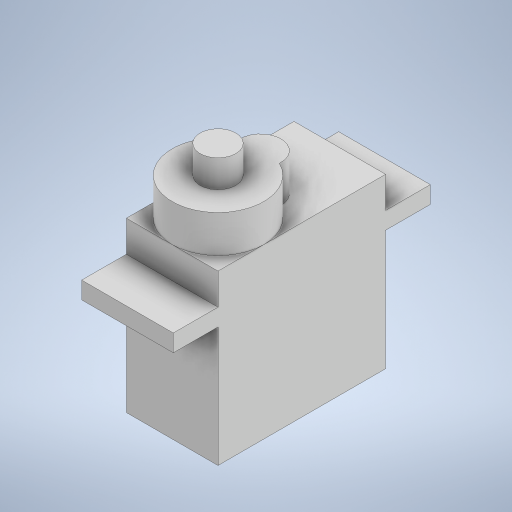
# Autodesk Inventor part: servomoteur
Saved by Autodesk Inventor 2024.1 (Build 281209000, 209)
## iProperties
Created: 2024-04-06
Part Number: servomoteur
Material: Générique
Document SubType Name: Modeling
Designer: chass
Density: 1 g/cm^3
Appearance: Par défaut
Author: chass
Autodesk Inventor part; units mm, degrees
ref_plane "YZ Plane" through (0, 0, 0) normal (1, 0, 0) x (0, 1, 0)
ref_plane "XZ Plane" through (0, 0, 0) normal (0, 1, 0) x (-1, 0, 0)
ref_plane "XY Plane" through (0, 0, 0) normal (0, 0, 1) x (1, 0, 0)
sketch "Esquisse1" plane through (0, 0, 0) normal (0, 1, 0) x (-1, 0, 0)
  line L0 (6.15, 11.25) -> (-6.15, 11.25)
  line L1 (-6.15, 11.25) -> (-6.15, -11.25)
  line L2 (-6.15, -11.25) -> (6.15, -11.25)
  line L3 (6.15, -11.25) -> (6.15, 11.25)
  line L4 (6.15, 11.25) -> (-6.15, -11.25)
  line L5 (-6.15, 11.25) -> (6.15, -11.25)
  point P0 (0, 0)
  point P1 (0, 0)
  point P2 (0, 0)
  dimension "d0" = 22.5
  dimension "d1" = 12.3
  constraints: 12 end point, 2 midpoint, 2 parallel, 1 coincident, 1 horizontal, 1 perpendicular
  measures "d0" distance of L2.end L0.start
  measures "d1" distance of L1.end L2.end
extrude "Extrusion1" add sketch "Esquisse1" along normal blind 22.6
sketch "Esquisse2" plane through (-6.15, 0, 11.25) normal (0, 0, 1) x (1, 0, 0)
  line L0 (0, 0) -> (0, 22.6) projected
  line L1 (12.3, 0) -> (12.3, 22.6) projected
  line L2 (0, 18.4) -> (12.3, 18.4)
  line L3 (12.3, 18.4) -> (12.3, 16.1)
  line L4 (12.3, 16.1) -> (0, 16.1)
  line L5 (0, 16.1) -> (0, 18.4)
  line L6 (0, 0) -> (12.3, 0) projected
  point P0 (6.15, 0)
  point P1 (0, 16.1)
  dimension "d4" = 2.3
  dimension "d5" = 16.1
  constraints: 8 end point, 2 parallel, 2 point on line, 1 horizontal, 1 perpendicular
  measures "d4" distance between parallel lines of L4 L2
  measures "d5" distance between parallel lines of L4 L6
extrude "Extrusion2" add sketch "Esquisse2" along normal blind 6 contours L0 L2 L1 L4
sketch "Esquisse3" plane through (6.15, 0, -11.25) normal (0, 0, -1) x (-1, 0, 0)
  line L0 (12.3, 18.4) -> (0, 18.4) projected
  line L1 (12.3, 0) -> (12.3, 16.1) projected
  line L2 (0, 18.4) -> (12.3, 18.4)
  line L3 (12.3, 18.4) -> (12.3, 16.1)
  line L4 (12.3, 16.1) -> (0, 16.1)
  line L5 (0, 16.1) -> (0, 18.4)
  point P0 (6.15, 0)
  constraints: 8 end point, 2 parallel, 1 horizontal, 1 perpendicular
extrude "Extrusion3" add sketch "Esquisse3" along normal blind 6
sketch "Esquisse4" plane through (0, 22.6, 0) normal (0, 1, 0) x (1, 0, 0)
  circle A0 centre (0, -5.1) radius 6.15
  line L0 (-6.15, 11.25) -> (-6.15, -11.25) projected
  line L1 (-6.15, -11.25) -> (6.15, -11.25) projected
  circle A1 centre (0, 0.6) radius 2.75
  point P0 (0, 0)
  point P1 (-2.743, 0.4044)
  point P2 (2.743, 0.4044)
  dimension "d10" = 12.3
  dimension "d11" = 6.15
  dimension "d12" = 5.5
  dimension "d13" = 14.6
  constraints: 2 centre point, 1 tangent
  measures "d10" diameter of A0
  measures "d11" distance from line of L1 A0.centre
  measures "d12" diameter of A1
extrude "Extrusion4" add sketch "Esquisse4" along normal blind 5 contours A0 A1 | A1 A0 | A0 A1
sketch "Esquisse5" plane through (0, 27.6, 0) normal (0, 1, 0) x (1, 0, 0)
  arc A0 (-6.15, -5.1) -> (0, -11.25) centre (0, -5.1) ccw projected
  circle A1 centre (0, -5.1) radius 2.4
  point P0 (0, 0)
  dimension "d16" = 4.8
  constraints: 1 centre point, 1 coincident
  measures "d16" diameter of A1
extrude "Extrusion5" add sketch "Esquisse5" along normal blind 3.7
